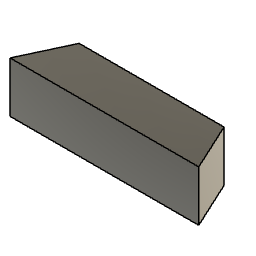
뎁스 사이즈 (Autodesk Fusion 360 design; units mm, degrees)
Autodesk Fusion 360 part; units mm, degrees
sketch "스케치1" plane through (0, 0, 0) normal (0, 0, 1) x (1, 0, 0)
  line L0 (107.5, 35) -> (-107.5, 35)
  line L1 (-107.5, 35) -> (-107.5, -35)
  line L2 (-107.5, -35) -> (107.5, -35)
  line L3 (107.5, -35) -> (107.5, 35)
  line L4 (107.5, 35) -> (-107.5, -35) construction
  line L5 (-107.5, 35) -> (107.5, -35) construction
  line L6 (0, -35) -> (140, -35)
  line L7 (0, -35) -> (-140, -35)
  line L8 (-140, -35) -> (-107.5, 35)
  line L9 (140, -35) -> (107.5, 35)
  dimension "d1" = 215
  dimension "d2" = 70
  dimension "d3" = 140
  dimension "d4" = 140
  constraint horizontal L0
  constraint perpendicular L0 L1
  constraint parallel L0 L2
  constraint parallel L1 L3
  constraint coincident L4 origin
  constraint coincident L5 origin
  constraint midpoint L2 L6.start
  constraint perpendicular L3 L6
  constraint parallel L2 L7
  measures "d1" distance of L1.end L2.end
  measures "d2" distance of L0.end L1.end
  measures "d3" distance of L6.start L6.end
  measures "d4" distance of L6.start L7.end
extrude "돌출1" add sketch "스케치1" along normal blind 75
